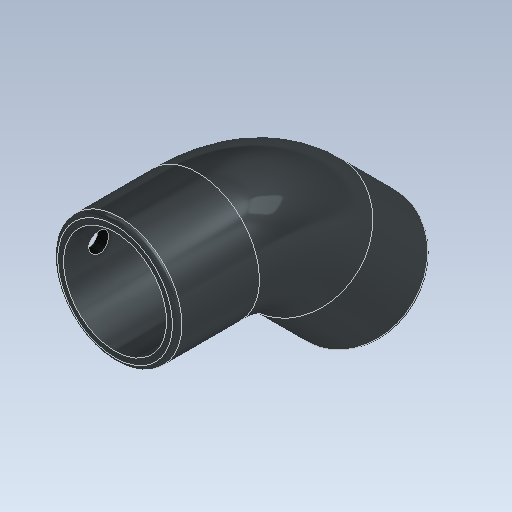
# Autodesk Inventor part: 55-7
Saved by Autodesk Inventor 2021 (Build 250183000, 183)
## iProperties
Created: 2020-04-23
Part Number: 55-7
Material: Iron, Cast
Document SubType Name: Modeling
Designer: Hannah
Density: 10.1598 g/cm^3
Appearance: Iron Gray
Mass: 810 g
Surface Area: 368.791 cm^2
Volume: 79.7261 cm^3
Catalog Web Link: https://keesystems.com/store/fittings/kee-klamp/55-obtuse-angle-elbow.html
Vendor: Kee Systems
Description: 120 to 150 deg elbow
Length: n/a
OD: n/a
Size: 7
Author: Hannah
Revision Number: -
Autodesk Inventor part; units mm, degrees
ref_plane "YZ Plane" through (0, 0, 0) normal (1, 0, 0) x (0, 1, 0)
ref_plane "XZ Plane" through (0, 0, 0) normal (0, 1, 0) x (-1, 0, 0)
ref_plane "XY Plane" through (0, 0, 0) normal (0, 0, 1) x (1, 0, 0)
sketch "Sketch3" plane through (0, 0, 0) normal (1, 0, 0) x (0, 1, 0)
  line L0 (0, 0) -> (0, -35.1472)
  line L1 (-17.5736, -77.5736) -> (-42.4264, -102.4264)
  arc A0 (-17.5736, -77.5736) -> (0, -35.1472) centre (-60, -35.1472) ccw
  point P0 (0, -60)
  point P1 (0, -15)
  point P2 (-31.8198, -91.8198)
  dimension "d34" = 60
  dimension "d35" = 60
  dimension "d36" = 135
  dimension "d37" = 60
  dimension "d40" = 15
  dimension "d41" = 15
  constraints: 4 end point, 4 point on line, 2 point on circle, 2 tangent, 1 centre point, 1 vertical
  measures "d34" distance of L0.start point (0, -60)
  measures "d35" distance of point (0, -60) L1.end
  measures "d36" angle of L1 L0
  measures "d37" radius of A0
  measures "d40" distance of point (-31.82, -91.82) L1.end
  measures "d41" distance of L0.start point (0, -15)
sketch "Sketch1" plane through (0, 0, 0) normal (0, 0, 1) x (1, 0, 0)
  circle A0 centre (0, 0) radius 22
  circle A1 centre (0, 0) radius 26.5
  dimension "d1" = 53
  dimension "d2" = 44
  constraints: 2 centre point, 2 coincident
  measures "d1" diameter of A1
  measures "d2" diameter of A0
sweep "Sweep1" add profiles "Sketch1" path "Sketch3" path curves L0 A0 L1
hole "Hole3" at (0, 0, -15) at (0, -31.8198, -91.8198) direction (-1, 0, 0) diameter 8.376 end through all
fillet "Fillet3" radius 2 2 edges at (-26.5, 0, 0) (-26.5, -42.4264, -102.4264)
body "Solid2"
